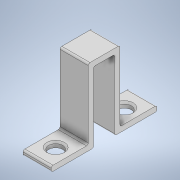
# Autodesk Inventor part: CLIP V1
Saved by Autodesk Inventor 2020 (Build 240168000, 168)
## iProperties
Created: 2023-12-19
Part Number: CLIP V1
Material: Generic
Document SubType Name: Modeling
Designer: HP
Density: 1 g/cm^3
Appearance: Default
Author: HP
Autodesk Inventor part; units mm, degrees
ref_plane "YZ Plane" through (0, 0, 0) normal (1, 0, 0) x (0, 1, 0)
ref_plane "XZ Plane" through (0, 0, 0) normal (0, 1, 0) x (-1, 0, 0)
ref_plane "XY Plane" through (0, 0, 0) normal (0, 0, 1) x (1, 0, 0)
sketch "Sketch1" plane through (0, 0, 0) normal (1, 0, 0) x (0, 1, 0)
  line L0 (0, 0) -> (0, -12)
  line L1 (0, -12) -> (20, -12)
  line L2 (20, -12) -> (20, -18)
  line L3 (20, -18) -> (0, -18)
  line L4 (0, -18) -> (0, -30)
  line L5 (1.5, 0) -> (1.5, -10.5)
  line L6 (1.5, -10.5) -> (21.5, -10.5)
  line L7 (21.5, -10.5) -> (21.5, -19.5)
  line L8 (21.5, -19.5) -> (1.5, -19.5)
  line L9 (1.5, -19.5) -> (1.5, -30)
  line L10 (1.5, 0) -> (0, 0)
  line L11 (1.5, -30) -> (0, -30)
  dimension "d0" = 12
  dimension "d1" = 12
  dimension "d2" = 6
  dimension "d3" = 20
  dimension "d4" = 1.5
  constraints: 24 end point, 6 perpendicular, 2 horizontal, 2 point on line, 1 coincident, 1 vertical, 4 other
  measures "d0" distance of L0.start L0.end
  measures "d1" distance of L3.end L4.end
  measures "d2" distance of L1.end L2.end
  measures "d3" distance between parallel lines of L4 L2
  measures "d4" distance between parallel lines of L1 L6
extrude "Extrusion1" add sketch "Sketch1" along normal blind 8
sketch "Sketch2" plane through (0, 1.5, 0) normal (0, 1, 0) x (1, 0, 0)
  line L0 (0, 0) -> (8, 0) construction
  line L1 (0, 10.5) -> (0, 0) construction
  line L2 (0, 30) -> (0, 19.5) construction
  point P0 (4, 5.25)
  point P1 (4, 24.75)
  point P2 (0, 5.25)
  point P3 (0, 24.75)
  point P4 (4, 0)
  point P5 (4, 0)
  constraints: 4 midpoint, 2 horizontal alignment, 2 vertical alignment
hole "Hole1" at (4, 1.5, -5.25) at (4, 1.5, -24.75) direction (0, -1, 0) diameter 4 end through all countersink diameter 5 countersink angle 90
fillet "Fillet1" radius 0.5 12 edges at (4, 21.5, -10.5) (4, 21.5, -19.5) (4, 20, -12) (4, 20, -18) (4, 0, -12) (4, 0, -18) (4, 1.5, -10.5) (4, 1.5, -19.5) (4, 1.5, -30) (4, 0, -30) (4, 1.5, 0) (4, 0, 0)
body "Solid1"
